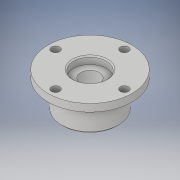
# Autodesk Inventor part: Фланец
Saved by Autodesk Inventor 2019 (Build 230136000, 136)
## iProperties
Created: 2020-04-06
Part Number: Фланец
Material: Типовые
Document SubType Name: Modeling
Designer: Diana
Density: 1 g/cm^3
Appearance: По умолчанию
Author: Diana
Autodesk Inventor part; units mm, degrees
ref_plane "YZ Plane" through (0, 0, 0) normal (1, 0, 0) x (0, 1, 0)
ref_plane "XZ Plane" through (0, 0, 0) normal (0, 1, 0) x (-1, 0, 0)
ref_plane "XY Plane" through (0, 0, 0) normal (0, 0, 1) x (1, 0, 0)
sketch "Эскиз1" plane through (0, 0, 0) normal (0, 1, 0) x (-1, 0, 0)
  circle A0 centre (0, 0) radius 56
  circle A1 centre (46, 0) radius 5.5
  circle A2 centre (0, 46) radius 5.5
  circle A3 centre (-46, 0) radius 5.5
  circle A4 centre (0, -46) radius 5.5
  dimension "d0" = 112
  dimension "d1" = 11
  dimension "d2" = 46
  dimension "d5" = 360
  constraints: 5 centre point, 1 coincident, 10 other
  measures "d0" diameter of A0
  measures "d1" diameter of A1
  measures "d2" distance of point (0, 0) A1.centre
extrude "Выдавливание1" add sketch "Эскиз1" along normal blind 10
sketch "Эскиз3" plane through (0, 10, 0) normal (0, 1, 0) x (1, 0, 0)
  circle A0 centre (0, 0) radius 22
  dimension "d9" = 44
  constraints: 1 centre point, 1 coincident
  measures "d9" diameter of A0
extrude "Выдавливание2" cut sketch "Эскиз3" against normal blind 10
sketch "Эскиз4" plane through (0, 0, 0) normal (0, -1, 0) x (1, 0, 0)
  circle A0 centre (0, 0) radius 38
  dimension "d12" = 76
  constraints: 1 centre point, 1 coincident
  measures "d12" diameter of A0
extrude "Выдавливание3" add sketch "Эскиз4" along normal blind 38
sketch "Эскиз5" plane through (0, -38, 0) normal (0, -1, 0) x (1, 0, 0)
  circle A0 centre (0, 0) radius 12.5
  dimension "d15" = 25
  constraints: 1 centre point, 1 coincident
  measures "d15" diameter of A0
extrude "Выдавливание4" cut sketch "Эскиз5" against normal through all
chamfer "Фаска1" distance 1.6 angle 45 1 edges at (-22, 10, 0)
chamfer "Фаска2" distance 2.5 angle 45 1 edges at (-38, -38, 0)
sketch "Эскиз6" plane through (0, -38, 0) normal (0, -1, 0) x (1, 0, 0)
  point P0 (0, 0)
  point P1 (0, -24)
  point P2 (0, 24)
  dimension "d24" = 24
  dimension "d25" = 48
  constraints: 2 vertical alignment
  measures "d24" distance of point (0, -24) point (0, 0)
  measures "d25" distance of point (0, 24) point (0, -24)
hole "Отверстие1" at (0, -38, -24) at (0, -38, 24) direction (0, 1, 0) diameter 8.376 depth 24 tip angle 120 thread size "M10x1.5" class "6H" standard "ISO Metric profile"
chamfer "Фаска3" distance 1.6 angle 45 2 edges at (0, -38, -19.812) (0, -38, 28.188)
